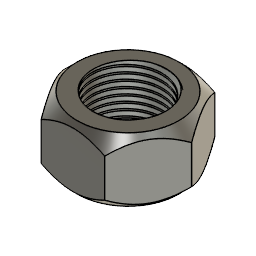
Hex nut (Autodesk Fusion 360 design; units mm, degrees)
part number: 2026-02-14-12-56-13-712
Autodesk Fusion 360 part; units mm, degrees
note: some values were not read from the file. Set by a fixed rule: the direction of a hole.
sketch "Sketch1" plane through (0, 0, 0) normal (0, 0, 1) x (1, 0, 0)
  line L0 (10, 0) -> (5, 8.6603)
  line L1 (5, 8.6603) -> (-5, 8.6603)
  line L2 (-5, 8.6603) -> (-10, 0)
  line L3 (-10, 0) -> (-5, -8.6603)
  line L4 (-5, -8.6603) -> (5, -8.6603)
  line L5 (5, -8.6603) -> (10, 0)
  dimension "d1" = 10
  measures "d1" distance of L0.start origin
extrude "Extrude1" add sketch "Sketch1" along normal blind 10
sketch "Sketch2" plane through (0, 0, 0) normal (0, 0, 1) x (1, 0, 0)
sketch "Sketch3" plane through (0, 0, 0) normal (0, 1, 0) x (1, 0, 0)
  line L0 (10, -10) -> (8, -10)
  line L1 (10, -10) -> (10, -8)
  line L2 (10, -8) -> (8, -10)
  dimension "d4" = 2
  dimension "d5" = 2
  constraint horizontal L0
  constraint perpendicular L0 L1
  measures "d4" distance of L0.start L0.end
  measures "d5" distance of L0.start L1.end
revolve "Revolve1" cut sketch "Sketch3" angle 360 about axis through (0, 0, 1.75) along (0, 0, 1)
ref_plane "WorkPlane1" through (0, 0, 5) normal (0, 0, 1) x (1, 0, 0)
mirror "Mirror1" about plane through (0, 0, 5) normal (0, 0, 1) of "Revolve1"
hole "Hole1" at (0, 0, 0) direction (0, 0, 1) diameter 11.035 depth 10 tip angle 180 countersink diameter 12 countersink angle 90
thread "Thread1" "GB Metric profile 12.0 M12x1 M12x1 6H" major diameter 12.152 minor diameter 11.035 pitch 1 angle 60 modelled right hand crest width 0.2719 on face at (0.275, 5.5106, 3.655) crest through (-5.5175, 0, 0.7325)
